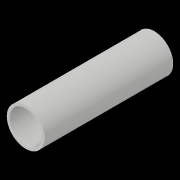
# Autodesk Inventor part: 3FT-SCH40-PVC
Saved by Autodesk Inventor 2022 (Build 260153000, 153)
## iProperties
Created: 2021-09-16
Part Number: 3FT-SCH40-PVC
Material: Generic
Document SubType Name: Modeling
Designer: timmy
Density: 1 g/cm^3
Appearance: Default
Author: timmy
Autodesk Inventor part; units mm, degrees
ref_plane "YZ Plane" through (0, 0, 0) normal (1, 0, 0) x (0, 1, 0)
ref_plane "XZ Plane" through (0, 0, 0) normal (0, 1, 0) x (-1, 0, 0)
ref_plane "XY Plane" through (0, 0, 0) normal (0, 0, 1) x (1, 0, 0)
sketch "Sketch1" plane through (0, 0, 0) normal (0, 1, 0) x (-1, 0, 0)
  circle A0 centre (0, 0) radius 44.45
  circle A1 centre (0, 0) radius 38.6334
  dimension "d0" = 88.9
  dimension "d1" = 77.2668
  constraints: 2 centre point, 2 coincident
  measures "d0" diameter of A0
  measures "d1" diameter of A1
extrude "Extrusion1" add sketch "Sketch1" along normal blind 304.8
ref_plane "Work Plane1" through (0, 304.8, 0) normal (0, 1, 0) x (1, 0, 0)
ref_plane "Work Plane3" through (0, 228.6, 0) normal (0, 1, 0) x (1, 0, 0)
ref_plane "Work Plane2" through (0, 152.4, 0) normal (0, 1, 0) x (1, 0, 0)
sketch "Sketch2" plane through (0, 304.8, 0) normal (0, 1, 0) x (1, 0, 0)
  line L0 (-49.0726, -48.8385) -> (49.0335, -48.8385)
  point P0 (0, 0)
  constraints: 2 end point, 1 horizontal
ref_plane "Work Plane4" through (-49.0726, 304.8, 48.8385) normal (0, 0, 1) x (1, 0, 0)
body "Solid1"
